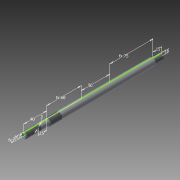
# Autodesk Inventor part: NagyTengely
Saved by Autodesk Inventor 2015 SP1 (Build 190203100, 203)
## iProperties
Created: 2014-08-10
Part Number: NagyTengely
Material: Generic
Document SubType Name: Modeling
Designer: laca
Density: 1 g/cm^3
Appearance: Default
Mass: 24.7061 g
Surface Area: 92.2611 cm^2
Volume: 24.7061 cm^3
Author: laca
Autodesk Inventor part; units mm, degrees
ref_plane "YZ Plane" through (0, 0, 0) normal (1, 0, 0) x (0, 1, 0)
ref_plane "XZ Plane" through (0, 0, 0) normal (0, 1, 0) x (-1, 0, 0)
ref_plane "XY Plane" through (0, 0, 0) normal (0, 0, 1) x (1, 0, 0)
sketch "Sketch1" plane through (0, 0, 0) normal (1, 0, 0) x (0, 1, 0)
  line L0 (0.5, 107.169868) -> (0.5, -132.830132)
  line L1 (0.5, -132.830132) -> (5.5, -132.830132)
  line L2 (5.5, -132.830132) -> (5.5, -117.830132)
  line L3 (5.5, -117.830132) -> (6.5, -117.830132)
  line L4 (6.5, -117.830132) -> (6.5, -42.830132)
  line L5 (6.5, -42.830132) -> (6.5, -42.830132)
  line L6 (6.5, -42.830132) -> (6.5, 7.169868)
  line L7 (6.5, 7.169868) -> (6.5, 7.169868)
  line L8 (6.5, 7.169868) -> (6.5, 67.169868)
  line L9 (6.5, 67.169868) -> (5.5, 67.169868)
  line L10 (5.5, 67.169868) -> (5.5, 107.169868)
  line L11 (5.5, 107.169868) -> (0.5, 107.169868)
  circle A0 centre (0.5, 82.169868) radius 1.5
  point P0 (0, 0)
  dimension "d2" = 5
  dimension "d3" = 5
  dimension "d4" = 6
  dimension "d5" = 6
  dimension "d6" = 6
  dimension "d7" = 40
  dimension "d8" = 50
  dimension "d9" = 60
  dimension "d10" = 75
  dimension "d11" = 15
  dimension "d28" = 3
  dimension "d43" = 15
  constraints: 24 end point, 10 perpendicular, 2 point on line, 2 vertical, 1 centre point
  measures "d2" distance between parallel lines of L0 L10
  measures "d3" distance of L0.end L1.end
  measures "d4" distance between parallel lines of L0 L4
  measures "d5" distance between parallel lines of L0 L8
  measures "d6" distance between parallel lines of L0 L6
  measures "d7" distance of L9.end L10.end
  measures "d8" distance of L5.end L6.end
  measures "d9" distance of L7.end L8.end
  measures "d10" distance of L3.end L4.end
  measures "d11" distance of L1.end L2.end
  measures "d28" diameter of A0
  measures "d43" vertical distance of L9.end A0.centre
sketch "Sketch1 outline for Revolution2" plane through (0, 0, 0) normal (1, 0, 0) x (0, 1, 0)
  line L0 (5.5, 107.169868) -> (0.5, 107.169868)
  line L1 (5.5, 67.169868) -> (5.5, 107.169868)
  line L2 (6.5, 67.169868) -> (5.5, 67.169868)
  line L3 (6.5, 7.169868) -> (6.5, 67.169868)
  line L4 (6.5, -42.830132) -> (6.5, 7.169868)
  line L5 (6.5, -117.830132) -> (6.5, -42.830132)
  line L6 (5.5, -117.830132) -> (6.5, -117.830132)
  line L7 (5.5, -132.830132) -> (5.5, -117.830132)
  line L8 (0.5, -132.830132) -> (5.5, -132.830132)
  line L9 (0.5, 107.169868) -> (0.5, -132.830132)
revolve "Revolution2" add sketch "Sketch1 outline for Revolution2" angle 360 about axis through (0, 0.5, 107.169868) along (0, 0, -1)
chamfer "Chamfer1" distance 1 angle 45 6 edges at (0, -4.5, 107.1699) (0, -5.5, 67.1699) (0, -5.5, 7.1699) (0, -5.5, -42.8301) (0, -5.5, -117.8301) (0, -4.5, -132.8301)
thread "Thread2" size "M12x1.5" class "6g" standard "ANSI Metric M Profile" length 20
thread "Thread3" size "M10x1" class "6g" standard "ANSI Metric M Profile" full length
sketch "Sketch1 outline for Extrusion2" plane through (0, 0, 0) normal (1, 0, 0) x (0, 1, 0)
  circle A0 centre (0.5, 82.169868) radius 1.5
extrude "Extrusion2" cut sketch "Sketch1 outline for Extrusion2" along normal through all both and the other way through all
thread "Thread4" size "M10x1.5" class "6g" standard "ANSI Metric M Profile" length 25
sketch "Sketch2" plane through (0, 0.5, 107.169868) normal (0, 0, 1) x (1, 0, 0)
  circle A0 centre (0, 0) radius 4 projected
  circle A1 centre (0, 0) radius 2.5
  point P0 (0, -0.5)
  dimension "d35" = 5
  constraints: 1 centre point, 1 coincident
  measures "d35" diameter of A1
sketch "Sketch2 outline for Extrusion3" plane through (0, 0.5, 107.169868) normal (0, 0, 1) x (1, 0, 0)
  circle A0 centre (0, 0) radius 2.5
extrude "Extrusion3" cut sketch "Sketch2 outline for Extrusion3" against normal blind 20
chamfer "Chamfer2" distance 1 angle 45 1 edges at (-2.5, 0.5, 107.1699)
thread "Thread5" size "M5x0.8" class "6H" standard "ANSI Metric M Profile" full length
equation "\"d6\" = d5"
equation "\"d10\" = NagyKerékSzélesege"
equation "\"ZártSzelvényFalVastagság\" = 1.5"
equation "\"ZártSzelvényBelsőÁtmérő\" = 12"
equation "\"ZártSzelvényKülsőÁtmérő\" = 15"
equation "\"CsapágyBelsőÁtmérő\" = 12"
equation "\"CsapágySzélesége\" = 8"
equation "\"CsapágyKülsőÁtmérő\" = 28"
equation "\"CsapágyHázBelsőÁtmérő\" = 26"
equation "\"CsapágyHázHoszza\" = 45"
equation "\"CsapágyHázKülsőÁtmérő\" = 32"
equation "\"NagyKerékSzélesege\" = 75"
body "Solid2"
